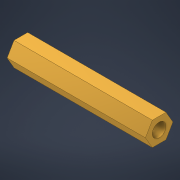
# Autodesk Inventor part: SpacerCamera
Saved by Autodesk Inventor 2022 (Build 260153000, 153)
## iProperties
Created: 2022-04-11
Part Number: SpacerCamera
Material: Brass, Soft Yellow
Document SubType Name: Modeling
Designer: ForseFire
Density: 8.47 g/cm^3
Appearance: Brass - Satin
Author: ForseFire
Autodesk Inventor part; units mm, degrees
ref_plane "YZ Plane" through (0, 0, 0) normal (1, 0, 0) x (0, 1, 0)
ref_plane "XZ Plane" through (0, 0, 0) normal (0, 1, 0) x (-1, 0, 0)
ref_plane "XY Plane" through (0, 0, 0) normal (0, 0, 1) x (1, 0, 0)
sketch "Sketch1" plane through (0, 0, 0) normal (1, 0, 0) x (0, 1, 0)
  line L0 (0, 3) -> (2.5981, 1.5)
  line L1 (2.5981, 1.5) -> (2.5981, -1.5)
  line L2 (2.5981, -1.5) -> (0, -3)
  line L3 (0, -3) -> (-2.5981, -1.5)
  line L4 (-2.5981, -1.5) -> (-2.5981, 1.5)
  line L5 (-2.5981, 1.5) -> (0, 3)
  circle A0 centre (0, 0) radius 1.5
  dimension "d0" = 6
  dimension "d1" = 3
  dimension "d4" = 5.1962
  constraints: 12 end point, 2 coincident, 1 centre point, 13 other
  measures "d0" distance of L2.end L0.start
  measures "d1" diameter of A0
  measures "d4" distance between parallel lines of L5 L2
extrude "Extrusion1" add sketch "Sketch1" along normal blind 30.296
body "Solid1"
